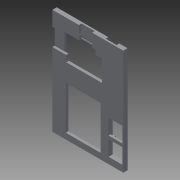
# Autodesk Inventor part: DisplayBottom2
Saved by Autodesk Inventor 2014 SP1 (Build 180222100, 222)
## iProperties
Created: 2014-03-24
Part Number: DisplayBottom2
Material: Generic
Document SubType Name: Modeling
Designer: patrigg
Density: 1 g/cm^3
Appearance: Default
Author: patrigg
Autodesk Inventor part; units mm, degrees
ref_plane "YZ Plane" through (0, 0, 0) normal (1, 0, 0) x (0, 1, 0)
ref_plane "XZ Plane" through (0, 0, 0) normal (0, 1, 0) x (-1, 0, 0)
ref_plane "XY Plane" through (0, 0, 0) normal (0, 0, 1) x (1, 0, 0)
sketch "Sketch2" plane through (0, 0, 0) normal (0, 1, 0) x (-1, 0, 0)
  line L0 (-33.5, -50) -> (33.5, -50)
  line L1 (33.5, -50) -> (33.5, 50)
  line L2 (33.5, 50) -> (-33.5, 50)
  line L3 (-33.5, 50) -> (-33.5, -50)
  line L4 (-33.5, -50) -> (33.5, 50) construction
  line L5 (33.5, -50) -> (-33.5, 50) construction
  point P0 (0, 0)
  dimension "d0" = 67
  dimension "d1" = 100
  constraints: 12 end point, 2 midpoint, 2 parallel, 1 horizontal, 1 perpendicular
  measures "d0" distance of L2.end L1.end
  measures "d1" distance of L1.end L0.end
extrude "Extrusion1" add sketch "Sketch2" along normal blind 4
sketch "Sketch3" plane through (0, 4, 0) normal (0, 1, 0) x (1, 0, 0)
  line L0 (33.5, 50) -> (-33.5, 50) projected
  line L1 (-23.5, -6.5) -> (14.5, -6.5)
  line L2 (14.5, -6.5) -> (14.5, 46)
  line L3 (14.5, 46) -> (-23.5, 46)
  line L4 (-23.5, 46) -> (-23.5, -6.5)
  line L5 (-23.5, -6.5) -> (14.5, 46) construction
  line L6 (14.5, -6.5) -> (-23.5, 46) construction
  line L7 (-33.5, 50) -> (-33.5, -50) projected
  point P0 (0, 0)
  point P1 (-4.5, 19.75)
  dimension "d4" = 38
  dimension "d5" = 52.5
  dimension "d6" = 4
  dimension "d111" = 10
  constraints: 12 end point, 2 midpoint, 2 parallel, 1 horizontal, 1 perpendicular
  measures "d4" distance of L3.end L2.end
  measures "d5" distance of L2.end L1.end
  measures "d6" distance between parallel lines of L0 L3
  measures "d111" distance between parallel lines of L4 L7
extrude "Extrusion2" cut sketch "Sketch3" against normal blind 1.5
sketch "Sketch4" plane through (0, 2.5, 0) normal (0, 1, 0) x (1, 0, 0)
  line L0 (14.5, -6.5) -> (-23.5, -6.5) projected
  line L1 (14.5, 46) -> (14.5, -6.5) projected
  line L2 (-23.5, 46) -> (14.5, 46) projected
  line L3 (-23.5, -6.5) -> (-23.5, 46) projected
  line L4 (-21, 44.5) -> (12, 44.5)
  line L5 (12, 44.5) -> (12, 3.5)
  line L6 (12, 3.5) -> (-21, 3.5)
  line L7 (-21, 3.5) -> (-21, 44.5)
  line L8 (-21, 44.5) -> (12, 3.5) construction
  line L9 (12, 44.5) -> (-21, 3.5) construction
  point P0 (0, 0)
  point P1 (-4.5, 24)
  dimension "d9" = 10
  dimension "d10" = 1.5
  dimension "d11" = 2.5
  dimension "d12" = 2.5
  constraints: 12 end point, 2 midpoint, 2 parallel, 1 horizontal, 1 perpendicular
  measures "d9" distance between parallel lines of L0 L6
  measures "d10" distance between parallel lines of L2 L4
  measures "d11" distance between parallel lines of L1 L5
  measures "d12" distance between parallel lines of L3 L7
extrude "Extrusion3" cut sketch "Sketch4" against normal blind 2.5 contours L4 L5 L6 L7
sketch "Sketch12" plane through (0, 4, 0) normal (0, 1, 0) x (1, 0, 0)
  line L0 (-24.5, -37.5) -> (13.5, -37.5)
  line L1 (13.5, -37.5) -> (13.5, -13.5)
  line L2 (13.5, -13.5) -> (-24.5, -13.5)
  line L3 (-24.5, -13.5) -> (-24.5, -37.5)
  line L4 (-24.5, -37.5) -> (13.5, -13.5) construction
  line L5 (13.5, -37.5) -> (-24.5, -13.5) construction
  line L6 (-23.5, -6.5) -> (-23.5, 46) projected
  line L7 (14.5, -6.5) -> (-23.5, -6.5) projected
  point P0 (0, 0)
  point P1 (-5.5, -25.5)
  point P2 (-5.5, -25.5)
  dimension "d58" = 38
  dimension "d59" = 24
  dimension "d112" = 1
  dimension "d154" = 7
  constraints: 12 end point, 3 midpoint, 2 parallel, 1 horizontal, 1 perpendicular
  measures "d58" distance of L2.end L1.end
  measures "d59" distance of L1.end L0.end
  measures "d112" distance between parallel lines of L3 L6
  measures "d154" distance between parallel lines of L7 L2
extrude "Extrusion10" cut sketch "Sketch12" against normal blind 4
sketch "Sketch18" plane through (13.5, 4, 13.5) normal (-1, 0, 0) x (0, 0, 1)
  line L0 (0, 0) -> (24, 0) projected
  line L1 (24, -4) -> (20, -4)
  line L2 (20, -4) -> (20, -1.8)
  line L3 (20, -1.8) -> (24, -1.8)
  line L4 (24, -1.8) -> (24, -4)
  point P0 (-13.5, -4)
  dimension "d88" = 4
  dimension "d89" = 1.8
  constraints: 8 end point, 2 parallel, 1 horizontal, 1 perpendicular
  measures "d88" distance of L2.end L3.end
  measures "d89" distance between parallel lines of L3 L0
extrude "Extrusion17" add sketch "Sketch18" along normal blind 6
sketch "Sketch20" plane through (-24.5, 4, 37.5) normal (1, 0, 0) x (0, 0, -1)
  line L0 (0, 0) -> (24, 0) projected
  line L1 (24, -4) -> (18, -4)
  line L2 (18, -4) -> (18, -1.8)
  line L3 (18, -1.8) -> (24, -1.8)
  line L4 (24, -1.8) -> (24, -4)
  point P0 (37.5, -4)
  dimension "d96" = 6
  dimension "d97" = 1.8
  constraints: 8 end point, 2 parallel, 1 horizontal, 1 perpendicular
  measures "d96" distance of L2.end L3.end
  measures "d97" distance between parallel lines of L3 L0
extrude "Extrusion19" add sketch "Sketch20" along normal blind 4
sketch "Sketch22" plane through (0, 0, 0) normal (0, -1, 0) x (1, 0, 0)
  line L0 (33.5, 50) -> (33.5, -50) projected
  line L1 (32.5, -44) -> (19.5, -44)
  line L2 (19.5, -44) -> (19.5, -12)
  line L3 (19.5, -12) -> (32.5, -12)
  line L4 (32.5, -12) -> (32.5, -44)
  line L5 (33.5, -50) -> (-33.5, -50) projected
  point P0 (0, 0)
  dimension "d102" = 1
  dimension "d103" = 13
  dimension "d110" = 32
  dimension "d155" = 6
  constraints: 8 end point, 2 parallel, 1 horizontal, 1 perpendicular
  measures "d102" distance between parallel lines of L4 L0
  measures "d103" distance between parallel lines of L2 L4
  measures "d110" distance between parallel lines of L3 L1
  measures "d155" distance between parallel lines of L5 L1
extrude "Extrusion21" cut sketch "Sketch22" against normal up to next
sketch "Sketch23" plane through (0, 4, 0) normal (0, 1, 0) x (1, 0, 0)
  line L0 (-24.5, -13.5) -> (13.5, -13.5) projected
  line L1 (14.5, 46) -> (14.5, -6.5) projected
  line L2 (14.5, -6.5) -> (-23.5, -6.5) projected
  line L3 (-23.5, -6.5) -> (-23.5, 46) projected
  line L4 (-21.5, -6.5) -> (-21.5, -13.5)
  line L5 (12.5, -6.5) -> (12.5, -13.5)
  point P0 (0, 0)
  dimension "d114" = 2
  dimension "d115" = 2
  constraints: 4 end point, 4 point on line, 2 perpendicular
  measures "d114" distance between parallel lines of L4 L3
  measures "d115" distance between parallel lines of L1 L5
extrude "Extrusion22" cut sketch "Sketch23" against normal up to surface (1.5 mm away)
sketch "Sketch24" plane through (32.5, 0, -44) normal (-1, 0, 0) x (0, 0, 1)
  line L0 (0, 0) -> (0, 4) projected
  line L1 (32, 0) -> (0, 0) projected
  line L2 (14.5, 0) -> (17.5, 0)
  line L3 (17.5, 0) -> (17.5, 2)
  line L4 (17.5, 2) -> (14.5, 2)
  line L5 (14.5, 2) -> (14.5, 0)
  line L6 (14.5, 0) -> (17.5, 2) construction
  line L7 (17.5, 0) -> (14.5, 2) construction
  point P0 (16, 1)
  dimension "d118" = 3
  dimension "d119" = 2
  dimension "d120" = 16
  constraints: 12 end point, 2 midpoint, 2 parallel, 1 collinear, 1 horizontal, 1 perpendicular
  measures "d118" distance of L4.end L3.end
  measures "d119" distance of L3.end L2.end
  measures "d120" distance from line of L0 point (16, 1)
extrude "Extrusion23" add sketch "Sketch24" along normal up to next
sketch "Sketch25" plane through (32.5, 2, -26.5) normal (0, 1, 0) x (1, 0, 0)
  line L0 (0, 0) -> (-13, 0) projected
  line L1 (0, 3) -> (-13, 3) projected
  line L2 (-8, 1) -> (-5, 1)
  line L3 (-5, 1) -> (-5, 3)
  line L4 (-5, 3) -> (-8, 3)
  line L5 (-8, 3) -> (-8, 1)
  line L6 (-8, 1) -> (-5, 3) construction
  line L7 (-5, 1) -> (-8, 3) construction
  point P0 (-32.5, -26.5)
  point P1 (-6.5, 2)
  point P2 (-6.5, 2)
  point P3 (-6.5, 0)
  dimension "d123" = 3
  dimension "d124" = 2
  constraints: 12 end point, 4 midpoint, 2 parallel, 1 collinear, 1 horizontal, 1 perpendicular, 1 vertical alignment
  measures "d123" distance of L4.end L3.end
  measures "d124" distance of L3.end L2.end
extrude "Extrusion24" cut sketch "Sketch25" against normal blind 0.5
fillet "Fillet6" radius 1 1 edges at (26, 1.5, -29.5)
sketch "Sketch26" plane through (32.5, 2, -26.5) normal (0, 1, 0) x (1, 0, 0)
  line L0 (0, 0) -> (-13, 0) projected
  line L1 (0, 3) -> (0, 0) projected
  circle A0 centre (-10.625, 1.5) radius 1.25
  circle A1 centre (-2.375, 1.5) radius 1.25
  point P0 (-32.5, -26.5)
  point P1 (-6.5, 1.5)
  point P2 (0, 1.5)
  point P3 (-6.5, 0)
  dimension "d128" = 2.5
  dimension "d129" = 2.5
  dimension "d130" = 4.125
  dimension "d131" = 8.25
  constraints: 3 horizontal alignment, 2 centre point, 2 midpoint, 1 vertical alignment
  measures "d128" diameter of A0
  measures "d129" diameter of A1
  measures "d130" distance of point (-6.5, 1.5) A0.centre
  measures "d131" distance of A1.centre A0.centre
extrude "Extrusion25" add sketch "Sketch26" along normal blind 2
chamfer "Chamfer3" distance 0.5 angle 45 2 edges at (28.875, 4, -28) (20.625, 4, -28)
sketch "Sketch27" plane through (0, 4, 0) normal (0, 1, 0) x (1, 0, 0)
  line L0 (-33.5, -50) -> (33.5, -50) projected
  line L1 (32.5, 12) -> (19.5, 12) projected
  line L2 (19.5, 44) -> (32.5, 44) projected
  line L3 (15.25, -50) -> (25.75, -50)
  line L4 (25.75, -50) -> (25.75, -32)
  line L5 (25.75, -32) -> (15.25, -32)
  line L6 (15.25, -32) -> (15.25, -50)
  line L7 (15.25, -50) -> (25.75, -32) construction
  line L8 (25.75, -50) -> (15.25, -32) construction
  line L9 (19.5, 12) -> (19.5, 44) projected
  line L10 (15.25, -42) -> (15.5, -42)
  line L11 (15.5, -42) -> (15.5, -32)
  line L12 (25.75, -42) -> (25.5, -42)
  line L13 (25.5, -42) -> (25.5, -32)
  point P0 (0, 0)
  point P1 (26, 44)
  point P2 (20.5, -41)
  point P3 (20.5, -41)
  point P4 (26, 12)
  dimension "d138" = 10.5
  dimension "d139" = 18
  dimension "d148" = 0.25
  dimension "d149" = 0.25
  dimension "d150" = 8
  dimension "d168" = 13
  constraints: 20 end point, 5 midpoint, 5 perpendicular, 4 point on line, 2 collinear, 2 parallel, 1 horizontal
  measures "d138" distance of L5.end L4.end
  measures "d139" distance of L4.end L3.end
  measures "d148" distance between parallel lines of L11 L6
  measures "d149" distance between parallel lines of L4 L13
  measures "d150" distance from line of L0 L10.end
  measures "d168" horizontal distance of L0.end point (20.5, -41)
extrude "Extrusion26" cut sketch "Sketch27" against normal blind 2.5 contours L6 L10 L11 L5 L13 L12 L4 L0
sketch "Sketch28" plane through (0, 4, 0) normal (0, 1, 0) x (1, 0, 0)
  line L0 (32.5, 12) -> (19.5, 12) projected
  line L1 (15.5, -32) -> (25.5, -32) projected
  line L2 (-33.5, -50) -> (15.25, -50) projected
  line L3 (24.75, 12) -> (24.75, -18.1789)
  line L4 (24.75, -18.1789) -> (18, -24.9289)
  line L5 (18, -24.9289) -> (18, -32)
  line L6 (27.25, 12) -> (27.25, -22.75)
  line L7 (27.25, -22.75) -> (23, -27)
  line L8 (23, -27) -> (23, -32)
  point P0 (0, 0)
  point P1 (20.5, -32)
  point P2 (20.5, -32)
  point P3 (26, 12)
  point P4 (26, 12)
  dimension "d170" = 2.5
  dimension "d171" = 5
  dimension "d172" = 135
  dimension "d173" = 135
  dimension "d174" = 2.5
  dimension "d175" = 1.25
  dimension "d176" = 5
  dimension "d177" = 5
  constraints: 12 end point, 4 point on line, 3 perpendicular, 2 coincident, 2 horizontal alignment, 2 midpoint, 1 parallel
  measures "d170" distance between parallel lines of L6 L3
  measures "d171" distance between parallel lines of L8 L5
  measures "d172" angle of L4 L5
  measures "d173" angle of L8 L7
  measures "d174" distance of L8.end point (20.5, -32)
  measures "d175" distance of L3.start point (26, 12)
  measures "d176" distance from line of L6.end L4
  measures "d177" distance of L8.end L7.end
extrude "Extrusion27" cut sketch "Sketch28" against normal blind 2.5
sketch "Sketch29" plane through (0, 0, 0) normal (0, -1, 0) x (1, 0, 0)
  line L0 (-24.5, 19.5) -> (-24.5, 37.5) projected
  line L1 (-24.5, 37.5) -> (7.5, 37.5) projected
  line L2 (-33.5, -50) -> (-33.5, 50) projected
  line L3 (-33.5, 50) -> (33.5, 50) projected
  line L4 (-24.5, 19.5) -> (-33.5, 19.5)
  line L5 (-24.5, 36) -> (-33.5, 36)
  point P0 (0, 0)
  dimension "d151" = 1.5
  constraints: 4 end point, 3 point on line, 1 parallel, 1 perpendicular
  measures "d151" distance between parallel lines of L1 L5
extrude "Extrusion28" cut sketch "Sketch29" against normal blind 2
sketch "Sketch30" plane through (0, 0, 0) normal (0, -1, 0) x (1, 0, 0)
  line L0 (-33.5, 50) -> (33.5, 50) projected
  line L1 (-8.5, 42) -> (4, 42)
  line L2 (4, 42) -> (4, 50)
  line L3 (4, 50) -> (-8.5, 50)
  line L4 (-8.5, 50) -> (-8.5, 42)
  line L5 (-8.5, 42) -> (4, 50) construction
  line L6 (4, 42) -> (-8.5, 50) construction
  line L7 (3.75, 37.5) -> (-8.25, 37.5)
  line L8 (-8.25, 37.5) -> (-8.25, 42)
  line L9 (-8.25, 42) -> (3.75, 42)
  line L10 (3.75, 42) -> (3.75, 37.5)
  line L11 (3.75, 37.5) -> (-8.25, 42) construction
  line L12 (-8.25, 37.5) -> (3.75, 42) construction
  line L13 (-24.5, 37.5) -> (7.5, 37.5) projected
  point P0 (0, 0)
  point P1 (-2.25, 46)
  point P2 (-2.25, 39.75)
  point P3 (-2.25, 39.75)
  point P4 (-2.25, 46)
  dimension "d156" = 12.5
  dimension "d157" = 8
  dimension "d158" = 16
  dimension "d162" = 12
  constraints: 24 end point, 6 midpoint, 4 parallel, 2 collinear, 2 horizontal, 2 perpendicular, 1 point on line, 1 vertical alignment
  measures "d156" distance of L3.end L2.end
  measures "d157" distance of L2.end L1.end
  measures "d158" distance from line of L4 L13.start
  measures "d162" distance between parallel lines of L8 L10
extrude "Extrusion29" cut sketch "Sketch30" against normal blind 2.5
chamfer "Chamfer5" distance 2 angle 45 2 edges at (24.75, 2.75, -12) (27.25, 2.75, -12)
fillet "Fillet8" radius 2 10 edges at (18, 2.75, 32) (18, 2.75, 24.9289) (23, 2.75, 32) (24.75, 2.75, 18.1789) (23, 2.75, 27) (27.25, 2.75, 22.75) (22.75, 2.75, -12) (24.75, 2.75, -10) (27.25, 2.75, -10) (29.25, 2.75, -12)
sketch "Sketch32" plane through (0, 2.5, 0) normal (0, -1, 0) x (1, 0, 0)
  line L0 (-8.25, 37.5) -> (-8.25, 42) projected
  line L1 (3.75, 37.5) -> (-8.25, 37.5) projected
  line L2 (3.75, 42) -> (3.75, 37.5) projected
  line L3 (-8.25, 42) -> (-8.5, 42) projected
  line L4 (-8.25, 38.5) -> (3.75, 38.5)
  point P0 (0, 0)
  dimension "d183" = 1
  constraints: 2 end point, 2 point on line, 1 parallel
  measures "d183" distance between parallel lines of L1 L4
extrude "Extrusion31" add sketch "Sketch32" along normal blind 0.5
body "Solid1"
